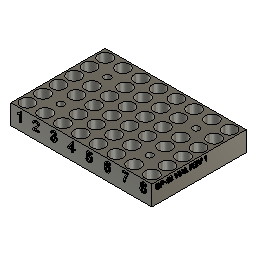
48_vial_plate v2 (Autodesk Fusion 360 design; units mm, degrees)
Autodesk Fusion 360 part; units mm, degrees
sketch "Sketch1" plane through (0, 0, 0) normal (0, 0, 1) x (1, 0, 0)
  line L0 (0, 0) -> (127.76, 0)
  line L1 (127.76, 0) -> (127.76, -85.48)
  line L2 (127.76, -85.48) -> (0, -85.48)
  line L3 (0, -85.48) -> (0, 0)
  dimension "d1" = 127.76
  dimension "d2" = 85.48
  constraint horizontal L0
  constraint vertical L1
  constraint horizontal L2
  constraint vertical L3
  constraint coincident L0.start L3.end
  measures "d1" distance of L0.start L0.end
  measures "d2" distance of L0.start L2.end
extrude "Extrude1" add sketch "Sketch1" along normal blind 18
sketch "Sketch2" plane through (0, 0, 18) normal (0, 0, 1) x (-1, 0, 0)
  line L0 (0, 85.48) -> (-127.76, 85.48)
  line L1 (-127.76, 85.48) -> (-127.76, 0)
  line L2 (-127.76, 0) -> (0, 0)
  line L3 (0, 0) -> (0, 85.48)
  point P0 (-7.5, 7.5)
  point P1 (-23.6086, 7.5)
  point P2 (-39.7171, 7.5)
  point P3 (-55.8257, 7.5)
  point P4 (-71.9343, 7.5)
  point P5 (-88.0429, 7.5)
  point P6 (-104.1514, 7.5)
  point P7 (-120.26, 7.5)
  point P8 (-7.5, 21.596)
  point P9 (-23.6086, 21.596)
  point P10 (-39.7171, 21.596)
  point P11 (-55.8257, 21.596)
  point P12 (-71.9343, 21.596)
  point P13 (-88.0429, 21.596)
  point P14 (-104.1514, 21.596)
  point P15 (-120.26, 21.596)
  point P16 (-7.5, 35.692)
  point P17 (-23.6086, 35.692)
  point P18 (-39.7171, 35.692)
  point P19 (-55.8257, 35.692)
  point P20 (-71.9343, 35.692)
  point P21 (-88.0429, 35.692)
  point P22 (-104.1514, 35.692)
  point P23 (-120.26, 35.692)
  point P24 (-7.5, 49.788)
  point P25 (-23.6086, 49.788)
  point P26 (-39.7171, 49.788)
  point P27 (-55.8257, 49.788)
  point P28 (-71.9343, 49.788)
  point P29 (-88.0429, 49.788)
  point P30 (-104.1514, 49.788)
  point P31 (-120.26, 49.788)
  point P32 (-7.5, 63.884)
  point P33 (-23.6086, 63.884)
  point P34 (-39.7171, 63.884)
  point P35 (-55.8257, 63.884)
  point P36 (-71.9343, 63.884)
  point P37 (-88.0429, 63.884)
  point P38 (-104.1514, 63.884)
  point P39 (-120.26, 63.884)
  point P40 (-7.5, 77.98)
  point P41 (-23.6086, 77.98)
  point P42 (-39.7171, 77.98)
  point P43 (-55.8257, 77.98)
  point P44 (-71.9343, 77.98)
  point P45 (-88.0429, 77.98)
  point P46 (-104.1514, 77.98)
  point P47 (-120.26, 77.98)
  dimension "d7" = -16.1086
  dimension "d8" = 14.096
hole "Hole1" at (7.5, -7.5, 18) at (23.6086, -7.5, 18) at (39.7171, -7.5, 18) at (55.8257, -7.5, 18) at (71.9343, -7.5, 18) at (88.0429, -7.5, 18) at (104.1514, -7.5, 18) at (120.26, -7.5, 18) at (7.5, -21.596, 18) at (39.7171, -21.596, 18) at (55.8257, -21.596, 18) at (71.9343, -21.596, 18) at (88.0429, -21.596, 18) at (120.26, -21.596, 18) at (120.26, -63.884, 18) at (7.5, -77.98, 18) at (7.5, -35.692, 18) at (7.5, -49.788, 18) at (7.5, -63.884, 18) at (120.26, -35.692, 18) at (55.8257, -35.692, 18) at (39.7171, -77.98, 18) at (88.0429, -35.692, 18) at (55.8257, -77.98, 18) at (23.6086, -35.692, 18) at (88.0429, -63.884, 18) at (39.7171, -49.788, 18) at (71.9343, -35.692, 18) at (120.26, -49.788, 18) at (88.0429, -77.98, 18) at (104.1514, -35.692, 18) at (88.0429, -49.788, 18) at (104.1514, -49.788, 18) at (120.26, -77.98, 18) at (71.9343, -77.98, 18) at (71.9343, -49.788, 18) at (104.1514, -77.98, 18) at (39.7171, -63.884, 18) at (23.6086, -49.788, 18) at (71.9343, -63.884, 18) at (55.8257, -49.788, 18) at (23.6086, -77.98, 18) at (39.7171, -35.692, 18) at (55.8257, -63.884, 18) direction (0, 0, -1) diameter 12 depth 13 tip angle 180
sketch "Sketch3" plane through (0, -85.48, 0) normal (0, -1, 0) x (1, 0, 0)
  line L0 (0, 0) -> (127.76, 0)
  line L1 (127.76, 0) -> (127.76, 18)
  line L2 (127.76, 18) -> (0, 18)
  line L3 (0, 18) -> (0, 0)
  line L4 (3.5565, 6.5495) -> (12.5565, 6.5495) construction
  line L5 (12.5565, 6.5495) -> (12.5565, 15.5495) construction
  line L6 (12.5565, 15.5495) -> (3.5565, 15.5495) construction
  line L7 (3.5565, 15.5495) -> (3.5565, 6.5495) construction
  line L8 (20.4645, 9.2162) -> (25.97, 9.2162) construction
  line L9 (25.97, 9.2162) -> (25.97, 15.6704) construction
  line L10 (25.97, 15.6704) -> (20.4645, 15.6704) construction
  line L11 (20.4645, 15.6704) -> (20.4645, 9.2162) construction
  line L12 (36.6034, 9.1401) -> (42.1089, 9.1401) construction
  line L13 (42.1089, 9.1401) -> (42.1089, 15.5943) construction
  line L14 (42.1089, 15.5943) -> (36.6034, 15.5943) construction
  line L15 (36.6034, 15.5943) -> (36.6034, 9.1401) construction
  line L16 (52.8422, 11.2891) -> (58.3477, 11.2891) construction
  line L17 (58.3477, 11.2891) -> (58.3477, 17.7434) construction
  line L18 (58.3477, 17.7434) -> (52.8422, 17.7434) construction
  line L19 (52.8422, 17.7434) -> (52.8422, 11.2891) construction
  line L20 (68.8728, 8.9033) -> (74.3783, 8.9033) construction
  line L21 (74.3783, 8.9033) -> (74.3783, 15.3576) construction
  line L22 (74.3783, 15.3576) -> (68.8728, 15.3576) construction
  line L23 (68.8728, 15.3576) -> (68.8728, 8.9033) construction
  line L24 (85.3408, 9.4502) -> (90.8463, 9.4502) construction
  line L25 (90.8463, 9.4502) -> (90.8463, 15.9045) construction
  line L26 (90.8463, 15.9045) -> (85.3408, 15.9045) construction
  line L27 (85.3408, 15.9045) -> (85.3408, 9.4502) construction
  line L28 (101.6723, 5.8436) -> (107.1778, 5.8437) construction
  line L29 (107.1778, 5.8437) -> (107.1776, 15.9765) construction
  line L30 (107.1776, 15.9765) -> (101.6721, 15.9764) construction
  line L31 (101.6721, 15.9764) -> (101.6723, 5.8436) construction
  line L32 (117.7723, 5.8436) -> (123.2778, 5.8437) construction
  line L33 (123.2778, 5.8437) -> (123.2776, 15.9765) construction
  line L34 (123.2776, 15.9765) -> (117.7721, 15.9764) construction
  line L35 (117.7721, 15.9764) -> (117.7723, 5.8436) construction
  dimension "d12" = 8
  dimension "d13" = 8
  dimension "d14" = 8
  dimension "d15" = 8
  dimension "d17" = 8
  dimension "d18" = 8
  dimension "d19" = 8
  dimension "d20" = 8
  text T0 "1" font "Arial" height 8 align centre top in box 9 x 9 at (3.5565, 6.5495) x (1, 0) y (0, 1) spacing 1 kerned
  text T1 "2" font "Arial" height 8 align centre top in box 5.5055 x 6.4543 at (20.4645, 9.2162) x (1, 0) y (0, 1) spacing 1 kerned
  text T2 "3" font "Arial" height 8 align centre top in box 5.5055 x 6.4543 at (36.6034, 9.1401) x (1, 0) y (0, 1) spacing 1 kerned
  text T3 "4" font "Arial" height 8 align centre top in box 5.5055 x 6.4543 at (52.8422, 11.2891) x (1, 0) y (0, 1) spacing 1 kerned
  text T4 "5" font "Arial" height 8 align centre top in box 5.5055 x 6.4543 at (68.8728, 8.9033) x (1, 0) y (0, 1) spacing 1 kerned
  text T5 "6\n" font "Arial" height 8 align centre top in box 5.5055 x 6.4543 at (85.3408, 9.4502) x (1, 0) y (0, 1) spacing 1 kerned
  text T6 "7\n" font "Arial" height 8 align centre top in box 5.5055 x 10.1328 at (101.6723, 5.8436) x (1, 0.000019) y (-0.000019, 1) spacing 1 kerned
  text T7 "8\n\n" font "Arial" height 8 align centre top in box 5.5055 x 10.1328 at (117.7723, 5.8436) x (1, 0.000019) y (-0.000019, 1) spacing 1 kerned
extrude "Extrude2" add sketch "Sketch3" along normal blind 1 text T0 T1 T2 T3 T4 T5 T6 T7
sketch "Sketch4" plane through (0, 0, 0) normal (-1, 0, 0) x (0, -1, 0)
  line L0 (0, 0) -> (85.48, 0)
  line L1 (85.48, 0) -> (85.48, 18)
  line L2 (85.48, 18) -> (0, 18)
  line L3 (0, 18) -> (0, 0)
  line L4 (4.0334, 6.1543) -> (10.2591, 6.1543) construction
  line L5 (10.2591, 6.1543) -> (10.2591, 15.4883) construction
  line L6 (10.2591, 15.4883) -> (4.0334, 15.4883) construction
  line L7 (4.0334, 15.4883) -> (4.0334, 6.1543) construction
  line L8 (18.5438, 3.9619) -> (24.7695, 3.9619) construction
  line L9 (24.7695, 3.9619) -> (24.7695, 13.2959) construction
  line L10 (24.7695, 13.2959) -> (18.5438, 13.2959) construction
  line L11 (18.5438, 13.2959) -> (18.5438, 3.9619) construction
  line L12 (32.5114, 6.0193) -> (38.7371, 6.0193) construction
  line L13 (38.7371, 6.0193) -> (38.7371, 15.3533) construction
  line L14 (38.7371, 15.3533) -> (32.5114, 15.3533) construction
  line L15 (32.5114, 15.3533) -> (32.5114, 6.0193) construction
  line L16 (32.5114, 6.0193) -> (38.7371, 6.0193) construction
  line L17 (38.7371, 6.0193) -> (38.7371, 15.3533) construction
  line L18 (38.7371, 15.3533) -> (32.5114, 15.3533) construction
  line L19 (32.5114, 15.3533) -> (32.5114, 6.0193) construction
  line L20 (46.6114, 6.0193) -> (52.8371, 6.0193) construction
  line L21 (52.8371, 6.0193) -> (52.8371, 15.3533) construction
  line L22 (52.8371, 15.3533) -> (46.6114, 15.3533) construction
  line L23 (46.6114, 15.3533) -> (46.6114, 6.0193) construction
  line L24 (60.4465, 4.2367) -> (66.6721, 4.2367) construction
  line L25 (66.6721, 4.2367) -> (66.6721, 13.5707) construction
  line L26 (66.6721, 13.5707) -> (60.4465, 13.5707) construction
  line L27 (60.4465, 13.5707) -> (60.4465, 4.2367) construction
  line L28 (74.5465, 4.2367) -> (80.7721, 4.2367) construction
  line L29 (80.7721, 4.2367) -> (80.7721, 13.5707) construction
  line L30 (80.7721, 13.5707) -> (74.5465, 13.5707) construction
  line L31 (74.5465, 13.5707) -> (74.5465, 4.2367) construction
  dimension "d23" = 8
  dimension "d24" = 8
  dimension "d25" = 8
  dimension "d26" = 8
  dimension "d27" = 8
  dimension "d28" = 8
  dimension "d29" = 8
  text T0 "A" font "Arial" height 8 align centre top in box 6.2257 x 9.334 at (4.0334, 6.1543) x (1, 0) y (0, 1) spacing 1 kerned
  text T1 "B" font "Arial" height 8 align centre top in box 6.2257 x 9.334 at (18.5438, 3.9619) x (1, 0) y (0, 1) spacing 1 kerned
  text T2 "C" font "Arial" height 8 align centre top in box 6.2257 x 9.334 at (32.5114, 6.0193) x (1, 0) y (0, 1) spacing 1 kerned
  text T3 "D" font "Arial" height 8 align centre top in box 6.2257 x 9.334 at (46.6114, 6.0193) x (1, 0) y (0, 1) spacing 1 kerned
  text T4 "E" font "Arial" height 8 align centre top in box 6.2257 x 9.334 at (60.4465, 4.2367) x (1, 0) y (0, 1) spacing 1 kerned
  text T5 "F" font "Arial" height 8 align centre top in box 6.2257 x 9.334 at (74.5465, 4.2367) x (1, 0) y (0, 1) spacing 1 kerned
extrude "Extrude3" add sketch "Sketch4" along normal blind 1 text T0 T1 T2 T3 T4 T5
sketch "Sketch5" plane through (127.76, 0, 0) normal (1, 0, 0) x (0, 1, 0)
  line L0 (-85.48, 0) -> (0, 0)
  line L1 (0, 0) -> (0, 18)
  line L2 (0, 18) -> (-85.48, 18)
  line L3 (-85.48, 18) -> (-85.48, 0)
  line L4 (-82.6452, 7.4287) -> (-35.8624, 7.5304) construction
  line L5 (-35.8624, 7.5304) -> (-35.8813, 16.2534) construction
  line L6 (-35.8813, 16.2534) -> (-82.6642, 16.1518) construction
  line L7 (-82.6642, 16.1518) -> (-82.6452, 7.4287) construction
  dimension "d32" = 4
  text T0 "BP 48 VIAL REV 1" font "Arial" height 4 align centre top in box 46.783 x 8.7231 at (-82.6452, 7.4287) x (0.999998, 0.002173) y (-0.002173, 0.999998) spacing 1
extrude "Extrude4" add sketch "Sketch5" along normal blind 1 text T0
sketch "Sketch6" plane through (0, 0, 18) normal (0, 0, 1) x (-1, 0, 0)
  circle A0 centre (-39.7171, 35.692) radius 6
  circle A1 centre (-55.8257, 49.788) radius 6
  circle A2 centre (-23.6086, 49.788) radius 6
  circle A3 centre (-104.1514, 77.98) radius 6
  circle A4 centre (-71.9343, 77.98) radius 6
  circle A5 centre (-104.1514, 49.788) radius 6
  circle A6 centre (-104.1514, 35.692) radius 6
  circle A7 centre (-120.26, 49.788) radius 6
  circle A8 centre (-39.7171, 49.788) radius 6
  circle A9 centre (-23.6086, 35.692) radius 6
  circle A10 centre (-88.0429, 35.692) radius 6
  circle A11 centre (-55.8257, 35.692) radius 6
  circle A12 centre (-7.5, 63.884) radius 6
  circle A13 centre (-7.5, 35.692) radius 6
  circle A14 centre (-120.26, 63.884) radius 6
  circle A15 centre (-88.0429, 21.596) radius 6
  circle A16 centre (-55.8257, 21.596) radius 6
  circle A17 centre (-7.5, 21.596) radius 6
  circle A18 centre (-104.1514, 7.5) radius 6
  circle A19 centre (-71.9343, 7.5) radius 6
  circle A20 centre (-39.7171, 7.5) radius 6
  circle A21 centre (-7.5, 7.5) radius 6
  circle A22 centre (-23.6086, 7.5) radius 6
  circle A23 centre (-55.8257, 7.5) radius 6
  circle A24 centre (-88.0429, 7.5) radius 6
  circle A25 centre (-120.26, 7.5) radius 6
  circle A26 centre (-39.7171, 21.596) radius 6
  circle A27 centre (-71.9343, 21.596) radius 6
  circle A28 centre (-120.26, 21.596) radius 6
  circle A29 centre (-7.5, 77.98) radius 6
  circle A30 centre (-7.5, 49.788) radius 6
  circle A31 centre (-120.26, 35.692) radius 6
  circle A32 centre (-39.7171, 77.98) radius 6
  circle A33 centre (-55.8257, 77.98) radius 6
  circle A34 centre (-88.0429, 63.884) radius 6
  circle A35 centre (-71.9343, 35.692) radius 6
  circle A36 centre (-88.0429, 77.98) radius 6
  circle A37 centre (-88.0429, 49.788) radius 6
  circle A38 centre (-120.26, 77.98) radius 6
  circle A39 centre (-71.9343, 49.788) radius 6
  circle A40 centre (-39.7171, 63.884) radius 6
  circle A41 centre (-71.9343, 63.884) radius 6
  circle A42 centre (-23.6086, 77.98) radius 6
  circle A43 centre (-55.8257, 63.884) radius 6
  line L0 (0, 85.48) -> (-127.76, 85.48)
  line L1 (-127.76, 85.48) -> (-127.76, 0)
  line L2 (-127.76, 0) -> (0, 0)
  line L3 (0, 0) -> (0, 85.48)
  point P0 (-104.1514, 63.884)
  point P1 (-104.1514, 21.596)
  point P2 (-23.6086, 21.596)
  point P3 (-23.6086, 63.884)
  constraint vertical P0 P1
  constraint horizontal P1 P2
  constraint vertical P2 P3
hole "Hole2" at (104.1514, -63.884, 18) at (104.1514, -21.596, 18) at (23.6086, -63.884, 18) at (23.6086, -21.596, 18) direction (0, 0, -1) diameter 3.4 depth 20 tip angle 180 counterbore diameter 6 counterbore depth 5
